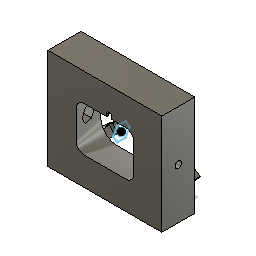
CameraMount v5 (Autodesk Fusion 360 design; units mm, degrees)
Autodesk Fusion 360 part; units mm, degrees
sketch "Sketch1" plane through (0, 0, 0) normal (0, 0, 1) x (1, 0, 0)
  line L0 (10, 0) -> (36, 0)
  line L1 (46, 10) -> (46, 30)
  line L2 (36, 40) -> (10, 40)
  line L3 (0, 30) -> (0, 10)
  arc A0 (10, 40) -> (0, 30) centre (10, 30) ccw
  arc A1 (46, 30) -> (36, 40) centre (36, 30) ccw
  arc A2 (0, 10) -> (10, 0) centre (10, 10) ccw
  arc A3 (36, 0) -> (46, 10) centre (36, 10) ccw
  line L4 (-7, 50) -> (-7, -10)
  line L5 (-7, -10) -> (53, -10)
  line L6 (53, -10) -> (53, 50)
  line L7 (53, 50) -> (-7, 50)
  point P0 (46, 40)
  point P1 (0, 40)
  dimension "d1" = 40
  dimension "d2" = 46
  dimension "d3" = 10
  dimension "d11" = 60
  dimension "d12" = 60
  dimension "d13" = 7
  dimension "d14" = 10
  constraint horizontal L0
  constraint vertical L1
  constraint horizontal L2
  constraint vertical L3
  constraint coincident P1 L3
  constraint coincident P1 L2
  constraint tangent L3 A0
  constraint tangent L2 A0
  constraint coincident P0 L2
  constraint coincident P0 L1
  constraint tangent L2 A1
  constraint tangent L1 A1
  constraint equal A0 A1
  constraint coincident origin L3
  constraint coincident origin L0
  constraint tangent L3 A2
  constraint tangent L0 A2
  constraint equal A0 A2
  constraint tangent L0 A3
  constraint tangent L1 A3
  constraint equal A0 A3
  constraint parallel L3 L4
  constraint parallel L0 L5
  constraint parallel L1 L6
  constraint parallel L2 L7
  measures "d1" distance of origin P1
  measures "d2" distance of P0 P1
  measures "d3" radius of A0
  measures "d11" distance of L4 L6
  measures "d12" distance of L5 L7
  measures "d13" distance of L1 L6
  measures "d14" distance of L2 L7
ref_plane "WorkPlane1" through (23, 20, 20) normal (0, 0, 1) x (1, 0, 0)
sketch "Sketch2" plane through (0, 0, 20) normal (0, 0, 1) x (1, 0, 0)
  arc A0 (40, 27) -> (35, 32) centre (35, 27) ccw
  line L0 (10, 32) -> (35, 32)
  arc A1 (10, 32) -> (5, 27) centre (10, 27) ccw
  line L1 (5, 10) -> (5, 27)
  arc A2 (5, 10) -> (10, 5) centre (10, 10) ccw
  line L2 (35, 5) -> (10, 5)
  arc A3 (35, 5) -> (40, 10) centre (35, 10) ccw
  line L3 (40, 27) -> (40, 10)
  arc A4 (10, 37) -> (0, 27) centre (10, 27) ccw
  line L4 (35, 37) -> (10, 37)
  arc A5 (45, 27) -> (35, 37) centre (35, 27) ccw
  line L5 (45, 10) -> (45, 27)
  arc A6 (35, 0) -> (45, 10) centre (35, 10) ccw
  line L6 (10, 0) -> (35, 0)
  arc A7 (0, 10) -> (10, 0) centre (10, 10) ccw
  line L7 (0, 27) -> (0, 10)
  line L8 (-12, 49) -> (-12, -12)
  line L9 (57, 49) -> (-12, 49)
  line L10 (-12, -12) -> (57, -12)
  line L11 (57, -12) -> (57, 49)
  constraint tangent A0 L3
  constraint tangent A3 L3
  constraint tangent A0 L0
  constraint tangent L0 A1
  constraint tangent A2 L2
  constraint tangent L1 A2
  constraint tangent A1 L1
  constraint tangent L2 A3
extrude "Extrude2" add sketch "Sketch2" against normal blind 20 contours A0 L0 A1 L1 A2 L2 A3 L3 | A4 L4 A5 L5 A6 L6 A7 L7 | L8 L9 L10 L11
loft "Loft3" cut profiles "Sketch2", "Sketch1" section 1 contours A0 L0 A1 L1 A2 L2 A3 L3 section 2 contours L0 L1 L2 L3 A0 A1 A2 A3
sketch "Sketch3" plane through (0, 0, 0) normal (0, 0, -1) x (-1, 0, 0)
  spline S0 degree 3 poles (-10, 40) (-9.0215, 40) (-7.771, 39.8444) (-6.4869, 39.3626) (-5.5317, 39.0042) (-4.5639, 38.4668) (-3.6996, 37.7656) (-2.4294, 36.7351) (-1.4076, 35.3459) (-0.7995, 33.918) (-0.2061, 32.5245) (0, 31.117) (0, 30) (0, 23.3333) (0, 16.6667) (0, 10) (0, 8.9531) (-0.1786, 7.652) (-0.6921, 6.3444) (-1.0742, 5.3717) (-1.639, 4.4014) (-2.3606, 3.5471) (-3.4213, 2.2914) (-4.8229, 1.3108) (-6.2289, 0.7383) (-7.601, 0.1796) (-8.956, 0) (-10, 0) (-18.6667, 0) (-27.3333, 0) (-36, 0) (-36.9785, 0) (-38.229, 0.1556) (-39.5131, 0.6374) (-40.4683, 0.9958) (-41.4361, 1.5332) (-42.3004, 2.2344) (-43.5706, 3.2649) (-44.5924, 4.6541) (-45.2005, 6.082) (-45.7939, 7.4755) (-46, 8.883) (-46, 10) (-46, 16.6667) (-46, 23.3333) (-46, 30) (-46, 31.0469) (-45.8214, 32.348) (-45.3079, 33.6556) (-44.9258, 34.6283) (-44.361, 35.5986) (-43.6394, 36.4529) (-42.5787, 37.7086) (-41.1771, 38.6892) (-39.7711, 39.2617) (-38.399, 39.8204) (-37.044, 40) (-36, 40) (-27.3333, 40) (-18.6667, 40) (-10, 40) knots 0 0 0 0 0.021708 0.021708 0.021708 0.037856 0.037856 0.037856 0.06159 0.06159 0.06159 0.084751 0.084751 0.084751 0.222983 0.222983 0.222983 0.244692 0.244692 0.244692 0.26084 0.26084 0.26084 0.284573 0.284573 0.284573 0.307734 0.307734 0.307734 0.5 0.5 0.5 0.521708 0.521708 0.521708 0.537856 0.537856 0.537856 0.56159 0.56159 0.56159 0.584751 0.584751 0.584751 0.722983 0.722983 0.722983 0.744692 0.744692 0.744692 0.76084 0.76084 0.76084 0.784573 0.784573 0.784573 0.807734 0.807734 0.807734 1 1 1 1
  line L0 (-57, 49) -> (-57, -12)
  line L1 (-57, -12) -> (12, -12)
  line L2 (12, -12) -> (12, 49)
  line L3 (12, 49) -> (-57, 49)
  line L4 (-70.1027, 51.994) -> (26.0629, -15.3419)
  line L5 (-55.7269, 51.9588) -> (11.1922, -14.9603)
  line L6 (-53.6358, -12.8693) -> (9.4959, 50.2625)
  line L7 (-60.6224, -8.3573) -> (16.8494, 45.8891)
  line L8 (-57, 49) -> (12, 49)
  line L9 (-53, 50) -> (7, 50)
  arc A0 (-42.0663, 38.2983) -> (-45.2036, 34.5594) centre (-22.2673, 18.4993) ccw
  arc A1 (-43.4805, 39.7125) -> (-46.8419, 35.7066) centre (-22.2673, 18.4993) ccw
  arc A2 (-44.8947, 41.1267) -> (-48.4802, 36.8537) centre (-22.2673, 18.4993) ccw
  arc A3 (0.6689, 34.5594) -> (-2.4683, 38.2983) centre (-22.2673, 18.4993) ccw
  arc A4 (2.3072, 35.7066) -> (-1.0541, 39.7125) centre (-22.2673, 18.4993) ccw
  arc A5 (3.9456, 36.8537) -> (-27.898, 50) centre (-22.2673, 18.4993) ccw
  arc A6 (0.3601, -4.1281) -> (3.9456, 0.1448) centre (-22.2673, 18.4993) ccw
  arc A7 (-46.8419, 1.292) -> (-43.4805, -2.7139) centre (-22.2673, 18.4993) ccw
  arc A8 (-1.0541, -2.7139) -> (2.3072, 1.292) centre (-22.2673, 18.4993) ccw
  arc A9 (-45.2036, 2.4391) -> (-42.0663, -1.2997) centre (-22.2673, 18.4993) ccw
  arc A10 (-2.4683, -1.2997) -> (0.6689, 2.4391) centre (-22.2673, 18.4993) ccw
  spline S1 degree 3 poles (-10, 32) (-15.9392, 32) (-29.0608, 32) (-35, 32) (-35.7154, 32) (-36.4305, 31.8441) (-37.081, 31.5464) (-37.7477, 31.2412) (-38.3457, 30.7873) (-38.8189, 30.2274) (-39.1409, 29.8464) (-39.4054, 29.4169) (-39.6007, 28.9579) (-39.8633, 28.3409) (-40, 27.6706) (-40, 27) (-40, 22.7299) (-40, 14.2701) (-40, 10) (-40, 9.2846) (-39.8441, 8.5695) (-39.5464, 7.919) (-39.2412, 7.2523) (-38.7873, 6.6543) (-38.2274, 6.1811) (-37.8464, 5.8591) (-37.4169, 5.5946) (-36.9579, 5.3993) (-36.3409, 5.1367) (-35.6706, 5) (-35, 5) (-29.0608, 5) (-15.9392, 5) (-10, 5) (-9.2846, 5) (-8.5695, 5.1559) (-7.919, 5.4536) (-7.2523, 5.7588) (-6.6543, 6.2127) (-6.1811, 6.7726) (-5.8591, 7.1536) (-5.5946, 7.5831) (-5.3993, 8.0421) (-5.1367, 8.6591) (-5, 9.3294) (-5, 10) (-5, 14.2701) (-5, 22.7299) (-5, 27) (-5, 27.7154) (-5.1559, 28.4305) (-5.4536, 29.081) (-5.7588, 29.7477) (-6.2127, 30.3457) (-6.7726, 30.8189) (-7.1536, 31.1409) (-7.5831, 31.4054) (-8.0421, 31.6007) (-8.6591, 31.8633) (-9.3294, 32) (-10, 32) knots -1 -1 -1 -1 -0.807734 -0.807734 -0.807734 -0.784573 -0.784573 -0.784573 -0.76084 -0.76084 -0.76084 -0.744692 -0.744692 -0.744692 -0.722983 -0.722983 -0.722983 -0.584751 -0.584751 -0.584751 -0.56159 -0.56159 -0.56159 -0.537856 -0.537856 -0.537856 -0.521708 -0.521708 -0.521708 -0.5 -0.5 -0.5 -0.307734 -0.307734 -0.307734 -0.284573 -0.284573 -0.284573 -0.26084 -0.26084 -0.26084 -0.244692 -0.244692 -0.244692 -0.222983 -0.222983 -0.222983 -0.084751 -0.084751 -0.084751 -0.06159 -0.06159 -0.06159 -0.037856 -0.037856 -0.037856 -0.021708 -0.021708 -0.021708 0 0 0 0
  line L10 (-10, 32) -> (-10, 40)
  spline S2 degree 3 poles (-10, 40) (-9.0215, 40) (-7.771, 39.8444) (-6.4869, 39.3626) (-5.5317, 39.0042) (-4.5639, 38.4668) (-3.6996, 37.7656) (-2.4294, 36.7351) (-1.4076, 35.3459) (-0.7995, 33.918) (-0.2061, 32.5245) (0, 31.117) (0, 30) (0, 23.3333) (0, 16.6667) (0, 10) (0, 8.9531) (-0.1786, 7.652) (-0.6921, 6.3444) (-1.0742, 5.3717) (-1.639, 4.4014) (-2.3606, 3.5471) (-3.4213, 2.2914) (-4.8229, 1.3108) (-6.2289, 0.7383) (-7.601, 0.1796) (-8.956, 0) (-10, 0) (-18.6667, 0) (-27.3333, 0) (-36, 0) (-36.9785, 0) (-38.229, 0.1556) (-39.5131, 0.6374) (-40.4683, 0.9958) (-41.4361, 1.5332) (-42.3004, 2.2344) (-43.5706, 3.2649) (-44.5924, 4.6541) (-45.2005, 6.082) (-45.7939, 7.4755) (-46, 8.883) (-46, 10) (-46, 16.6667) (-46, 23.3333) (-46, 30) (-46, 31.0469) (-45.8214, 32.348) (-45.3079, 33.6556) (-44.9258, 34.6283) (-44.361, 35.5986) (-43.6394, 36.4529) (-42.5787, 37.7086) (-41.1771, 38.6892) (-39.7711, 39.2617) (-38.399, 39.8204) (-37.044, 40) (-36, 40) (-27.3333, 40) (-18.6667, 40) (-10, 40) knots 0 0 0 0 0.021708 0.021708 0.021708 0.037856 0.037856 0.037856 0.06159 0.06159 0.06159 0.084751 0.084751 0.084751 0.222983 0.222983 0.222983 0.244692 0.244692 0.244692 0.26084 0.26084 0.26084 0.284573 0.284573 0.284573 0.307734 0.307734 0.307734 0.5 0.5 0.5 0.521708 0.521708 0.521708 0.537856 0.537856 0.537856 0.56159 0.56159 0.56159 0.584751 0.584751 0.584751 0.722983 0.722983 0.722983 0.744692 0.744692 0.744692 0.76084 0.76084 0.76084 0.784573 0.784573 0.784573 0.807734 0.807734 0.807734 1 1 1 1
  line L11 (-10, 40) -> (-10, 32)
  line L12 (-22.2673, 40) -> (-22.2673, 0)
  line L13 (-46, 18.4993) -> (0, 18.4993)
  arc A11 (-48.4802, 0.1448) -> (-44.8947, -4.1281) centre (-22.2673, 18.4993) ccw
  arc A12 (-31.952, -12) -> (-12.5826, -12) centre (-22.2673, 18.4993) ccw
  arc A13 (-50.2037, -1.062) -> (5.6691, -1.062) centre (-22.2673, 18.4993) ccw
  arc A14 (5.6691, 38.0606) -> (-50.2037, 38.0606) centre (-22.2673, 18.4993) ccw
  point P0 (-53, 50)
  dimension "d15" = 60
  dimension "d20" = 135
  dimension "d21" = 145
  dimension "d22" = 135
  dimension "d23" = 145
  constraint coincident A0.centre L4
  constraint coincident A0.centre L5
  constraint coincident A0.centre L7
  constraint coincident A0.centre L6
  constraint midpoint A0.centre L5
  constraint concentric A7 A9
  constraint coincident L4 A0.end
  constraint coincident L7 A9.start
  constraint coincident L4 A1.end
  constraint coincident L7 A7.start
  constraint coincident L4 A2.end
  constraint coincident L7 A11.start
  constraint coincident L6 A3.end
  constraint coincident L5 A0.start
  constraint concentric A0 A9
  constraint coincident L6 A4.end
  constraint coincident L5 A1.start
  constraint concentric A1 A7
  constraint coincident L9 A5.end
  constraint coincident L5 A2.start
  constraint concentric A2 A11
  constraint coincident L4 A10.end
  constraint coincident L7 A3.start
  constraint concentric A3 A9
  constraint coincident L4 A8.end
  constraint coincident L7 A4.start
  constraint concentric A4 A7
  constraint coincident L4 A6.end
  constraint coincident L7 A5.start
  constraint concentric A5 A11
  constraint coincident L1 A12.end
  constraint coincident L5 A6.start
  constraint concentric A6 A11
  constraint coincident L6 A7.end
  constraint coincident L5 A8.start
  constraint concentric A7 A8
  constraint coincident L6 A9.end
  constraint coincident L5 A10.start
  constraint concentric A9 A10
  constraint coincident S2 L12.start
  constraint coincident S2 L12.end
  constraint vertical L12
  constraint coincident S2 L13.start
  constraint coincident S2 L13.end
  constraint horizontal L13
  constraint coincident L6 A11.end
  constraint coincident L1 A12.start
  constraint concentric A11 A12
  constraint concentric A2 A13
  constraint coincident L4 A14.end
  constraint coincident L7 A13.start
  constraint coincident L4 A13.end
  constraint coincident L7 A14.start
  constraint concentric A13 A14
  measures "d15" diameter of A7
  measures "d20" angle of L5 L9
  measures "d21" angle of L4 L9
  measures "d22" angle of L6 L9
  measures "d23" angle of L7 L9
extrude "Extrude3" add sketch "Sketch3" along normal blind 10 contours L6 L7 A7 A9 | L4 L5 A8 A10 | L6 L7 A7 A11 | L4 L5 A6 A8 | L6 L7 A11 A13 | L4 L5 A6 A13
ref_plane "WorkPlane2" through (46.135, -1.5884, -8) normal (0, 0, -1) x (-1, 0, 0)
sketch "Sketch4" plane through (45.2732, -0.8445, -8) normal (0, 0, -1) x (1, 0, 0)
  arc A0 (-0.0697, -3.2836) -> (-3.2069, 0.4552) centre (-23.0059, -19.3438) ccw
  line L0 (-47.1212, 4.7715) -> (-42.8049, 0.4552)
  arc A1 (-42.8049, 0.4552) -> (-45.9422, -3.2836) centre (-23.0059, -19.3438) ccw
  line L1 (-45.9422, -3.2836) -> (-50.9424, 0.2175)
  line L2 (-3.2069, 0.4552) -> (1.1093, 4.7715)
  line L3 (4.9305, 0.2175) -> (-0.0697, -3.2836)
  spline S0 degree 3 poles (-35.2732, -40.8445) (-36.2518, -40.8445) (-37.5023, -40.6889) (-38.7864, -40.2071) (-39.7416, -39.8487) (-40.7094, -39.3113) (-41.5736, -38.6101) (-42.8438, -37.5796) (-43.8657, -36.1904) (-44.4737, -34.7625) (-45.0672, -33.369) (-45.2732, -31.9615) (-45.2732, -30.8445) (-45.2732, -24.1778) (-45.2732, -17.5112) (-45.2732, -10.8445) (-45.2732, -9.7975) (-45.0947, -8.4965) (-44.5811, -7.1889) (-44.1991, -6.2161) (-43.6343, -5.2459) (-42.9126, -4.3916) (-41.852, -3.1359) (-40.4504, -2.1553) (-39.0443, -1.5828) (-37.6722, -1.0241) (-36.3172, -0.8445) (-35.2732, -0.8445) (-26.6066, -0.8445) (-17.9399, -0.8445) (-9.2732, -0.8445) (-8.2947, -0.8445) (-7.0442, -1.0001) (-5.7601, -1.4819) (-4.8049, -1.8403) (-3.8371, -2.3777) (-2.9729, -3.0788) (-1.7026, -4.1094) (-0.6808, -5.4986) (-0.0727, -6.9265) (0.5207, -8.32) (0.7268, -9.7275) (0.7268, -10.8445) (0.7268, -17.5112) (0.7268, -24.1778) (0.7268, -30.8445) (0.7268, -31.8914) (0.5482, -33.1925) (0.0346, -34.5001) (-0.3474, -35.4728) (-0.9122, -36.4431) (-1.6339, -37.2974) (-2.6945, -38.5531) (-4.0961, -39.5337) (-5.5021, -40.1062) (-6.8742, -40.6649) (-8.2292, -40.8445) (-9.2732, -40.8445) (-17.9399, -40.8445) (-26.6066, -40.8445) (-35.2732, -40.8445) knots 0 0 0 0 0.021708 0.021708 0.021708 0.037856 0.037856 0.037856 0.06159 0.06159 0.06159 0.084751 0.084751 0.084751 0.222983 0.222983 0.222983 0.244692 0.244692 0.244692 0.26084 0.26084 0.26084 0.284573 0.284573 0.284573 0.307734 0.307734 0.307734 0.5 0.5 0.5 0.521708 0.521708 0.521708 0.537856 0.537856 0.537856 0.56159 0.56159 0.56159 0.584751 0.584751 0.584751 0.722983 0.722983 0.722983 0.744692 0.744692 0.744692 0.76084 0.76084 0.76084 0.784573 0.784573 0.784573 0.807734 0.807734 0.807734 1 1 1 1
  line L4 (11.7268, -49.8445) -> (11.7268, 11.1555)
  line L5 (11.7268, 11.1555) -> (-57.2732, 11.1555)
  line L6 (-57.2732, 11.1555) -> (-57.2732, -49.8445)
  line L7 (-57.2732, -49.8445) -> (11.7268, -49.8445)
  circle A2 centre (-23.0059, -19.3438) radius 31
  arc A3 (4.9305, 0.2175) -> (1.1093, 4.7715) centre (-23.0059, -19.3438) ccw
  arc A4 (-47.1212, 4.7715) -> (-50.9424, 0.2175) centre (-23.0059, -19.3438) ccw
  dimension "d27" = 62
  constraint concentric A0 A2
  measures "d27" diameter of A2
extrude "Extrude4" cut sketch "Sketch4" against normal blind 2 contours A0 L0 A1 L1 L2 L3 L5 L7 A2 | A0 L2 L3 A2 | L5 A2 | L7 A2 | L0 A1 L1 A2
fillet "Fillet1" radius 2 8 edges at (48.3926, -3.4224, 0) (-3.8579, -3.4224, 0) (44.2244, -3.4578, 0) (0.3102, -3.4578, 0) (-3.169, 0.6886, 0) (0.8181, 0.5012, 0) (43.7166, 0.5012, 0) (47.7037, 0.6886, 0)
ref_plane "WorkPlane3" through (10, 32, 20) normal (0, -0.928477, -0.371391) x (1, 0, 0)
sketch "Sketch5" plane through (10, 32, 20) normal (0, -0.928477, -0.371391) x (1, 0, 0)
  spline S0 degree 3 poles (0, 0) (5.9392, 0) (19.0608, 0) (25, 0) (25.7154, 0) (26.4305, 0.0579) (27.081, 0.1685) (27.7477, 0.2818) (28.3457, 0.4504) (28.8189, 0.6583) (29.1409, 0.7998) (29.4054, 0.9593) (29.6007, 1.1298) (29.8633, 1.359) (30, 1.6079) (30, 1.857) (30, 3.4428) (30, 6.5847) (30, 8.1706) (30, 8.4363) (29.8441, 8.7019) (29.5464, 8.9435) (29.2412, 9.191) (28.7873, 9.4132) (28.2274, 9.5889) (27.8464, 9.7085) (27.4169, 9.8067) (26.9579, 9.8793) (26.3409, 9.9768) (25.6706, 10.0275) (25, 10.0275) (19.0608, 10.0275) (5.9392, 10.0275) (0, 10.0275) (-0.7154, 10.0275) (-1.4305, 9.9697) (-2.081, 9.8591) (-2.7477, 9.7457) (-3.3457, 9.5772) (-3.8189, 9.3692) (-4.1409, 9.2277) (-4.4054, 9.0682) (-4.6007, 8.8977) (-4.8633, 8.6686) (-5, 8.4196) (-5, 8.1706) (-5, 6.5847) (-5, 3.4428) (-5, 1.857) (-5, 1.5912) (-4.8441, 1.3257) (-4.5464, 1.0841) (-4.2412, 0.8365) (-3.7873, 0.6144) (-3.2274, 0.4386) (-2.8464, 0.3191) (-2.4169, 0.2208) (-1.9579, 0.1483) (-1.3409, 0.0508) (-0.6706, 0) (0, 0) knots -1 -1 -1 -1 -0.807734 -0.807734 -0.807734 -0.784573 -0.784573 -0.784573 -0.76084 -0.76084 -0.76084 -0.744692 -0.744692 -0.744692 -0.722983 -0.722983 -0.722983 -0.584751 -0.584751 -0.584751 -0.56159 -0.56159 -0.56159 -0.537856 -0.537856 -0.537856 -0.521708 -0.521708 -0.521708 -0.5 -0.5 -0.5 -0.307734 -0.307734 -0.307734 -0.284573 -0.284573 -0.284573 -0.26084 -0.26084 -0.26084 -0.244692 -0.244692 -0.244692 -0.222983 -0.222983 -0.222983 -0.084751 -0.084751 -0.084751 -0.06159 -0.06159 -0.06159 -0.037856 -0.037856 -0.037856 -0.021708 -0.021708 -0.021708 0 0 0 0
  line L0 (0, 0) -> (0, -21.5407)
  spline S1 degree 3 poles (34.7657, -8.6115) (34.9276, -8.7211) (35.0725, -8.8322) (35.2005, -8.9438) (35.7939, -9.4614) (36, -9.9841) (36, -10.3989) (36, -12.8749) (36, -15.3508) (36, -17.8268) (36, -18.2156) (35.8214, -18.6988) (35.3079, -19.1844) (34.9258, -19.5457) (34.361, -19.906) (33.6394, -20.2233) (32.5787, -20.6896) (31.1771, -21.0538) (29.7711, -21.2665) (28.399, -21.4739) (27.044, -21.5407) (26, -21.5407) (17.3333, -21.5407) (8.6667, -21.5407) (0, -21.5407) knots 0.556595 0.556595 0.556595 0.556595 0.56159 0.56159 0.56159 0.584751 0.584751 0.584751 0.722983 0.722983 0.722983 0.744692 0.744692 0.744692 0.76084 0.76084 0.76084 0.784573 0.784573 0.784573 0.807734 0.807734 0.807734 1 1 1 1
  spline S2 degree 3 poles (34.6948, -8.5682) (34.7075, -8.5751) (34.7203, -8.5826) (34.744, -8.5972) (34.7548, -8.6042) (34.7657, -8.6115) knots -0.343561 -0.343561 -0.343561 -0.343561 -0.335497 -0.335497 -0.328702 -0.328702 -0.328702 -0.328702
  spline S3 degree 3 poles (33.1457, -7.8008) (33.5792, -7.9645) (33.9907, -8.1555) (34.4784, -8.4323) (34.5896, -8.4997) (34.6948, -8.5682) knots -1.903365 -1.903365 -1.903365 -1.903365 -1.702016 -1.702016 -1.63823 -1.63823 -1.63823 -1.63823
  spline S4 degree 3 poles (0, -21.5407) (-0.9785, -21.5407) (-2.229, -21.4829) (-3.5131, -21.3039) (-4.4683, -21.1708) (-5.4361, -20.9713) (-6.3004, -20.7108) (-7.5706, -20.3281) (-8.5924, -19.8122) (-9.2005, -19.2819) (-9.7939, -18.7643) (-10, -18.2416) (-10, -17.8268) (-10, -15.3508) (-10, -12.8749) (-10, -10.3989) (-10, -10.0101) (-9.8214, -9.5269) (-9.3079, -9.0413) (-8.9258, -8.68) (-8.361, -8.3197) (-7.6394, -8.0024) (-6.5787, -7.536) (-5.1771, -7.1719) (-3.7711, -6.9592) (-2.399, -6.7517) (-1.044, -6.685) (0, -6.685) (8.6667, -6.685) (17.3333, -6.685) (26, -6.685) (26.9785, -6.685) (28.229, -6.7428) (29.5131, -6.9218) (30.4683, -7.0549) (31.4361, -7.2544) (32.3004, -7.5149) (32.5953, -7.6037) (32.8786, -7.6995) (33.1457, -7.8008) knots 0 0 0 0 0.021708 0.021708 0.021708 0.037856 0.037856 0.037856 0.06159 0.06159 0.06159 0.084751 0.084751 0.084751 0.222983 0.222983 0.222983 0.244692 0.244692 0.244692 0.26084 0.26084 0.26084 0.284573 0.284573 0.284573 0.307734 0.307734 0.307734 0.5 0.5 0.5 0.521708 0.521708 0.521708 0.537856 0.537856 0.537856 0.543367 0.543367 0.543367 0.543367
  line L1 (0, -21.5407) -> (0, 0)
  line L2 (16, -24) -> (14, -24)
  line L3 (14, -24) -> (14, 20)
  line L4 (14, 20) -> (16, 20)
  line L5 (16, 20) -> (16, -24)
  constraint horizontal L2
  constraint vertical L3
  constraint horizontal L4
  constraint vertical L5
extrude "Extrude5" cut sketch "Sketch5" along normal blind -2 and the other way blind 0 contours S0 S4 L3 L5 | S1 S4 L3 L5 | S1 L2 L3 L5
fillet "Fillet2" radius 0.5 10 edges at (26, 36, 10) (26, 38.1541, 10) (24, 36, 10) (24, 38.1541, 10) (25, 42.1541, 0) (26, 41.077, 0) (24, 41.077, 0) (26, 33.077, 20) (25, 34.1541, 20) (24, 33.077, 20)
ref_plane "WorkPlane4" through (22.5, 18.5, 10) normal (1, 0, 0) x (0, -1, 0)
sketch "Sketch6" plane through (22.5, 18.5, 10) normal (1, 0, 0) x (0, 0, -1)
  line L0 (-5, 0) -> (-2.5, -4.3301)
  line L1 (-2.5, -4.3301) -> (2.5, -4.3301)
  line L2 (2.5, -4.3301) -> (5, 0)
  line L3 (5, 0) -> (2.5, 4.3301)
  line L4 (2.5, 4.3301) -> (-2.5, 4.3301)
  line L5 (-2.5, 4.3301) -> (-5, 0)
  circle A0 centre (0, 0) radius 2
  dimension "d38" = 5
  constraint coincident A0.centre origin
  measures "d38" distance of L0.start A0.centre
extrude "Extrude6" cut sketch "Sketch6" along normal mid plane 60 contours L0 L1 L2 L3 L4 L5 | A0
extrude "Extrude7" cut sketch "Sketch6" along normal mid plane 100 contours A0
